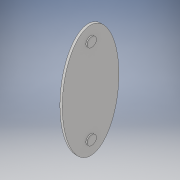
# Autodesk Inventor part: belt for lift
Saved by Autodesk Inventor 2017 (Build 210142000, 142)
## iProperties
Created: 2017-11-11
Part Number: belt for lift
Material: Generic
Document SubType Name: Modeling
Designer: User
Density: 1 g/cm^3
Appearance: Default
Author: User
Autodesk Inventor part; units mm, degrees
ref_plane "YZ Plane" through (0, 0, 0) normal (1, 0, 0) x (0, 1, 0)
ref_plane "XZ Plane" through (0, 0, 0) normal (0, 1, 0) x (-1, 0, 0)
ref_plane "XY Plane" through (0, 0, 0) normal (0, 0, 1) x (1, 0, 0)
sketch "Sketch1" plane through (0, 0, 0) normal (1, 0, 0) x (0, 1, 0)
  ellipse E0 centre (0, 0) end of major axis (76.2, 0) minor radius 38.1
  dimension "d0" = 38.1
  dimension "d1" = 76.2
  constraints: 1 coincident, 2 other
extrude "Extrusion1" add sketch "Sketch1" along normal blind 3.175
sketch "Sketch2" plane through (3.175, 0, 0) normal (1, 0, 0) x (0, 0, -1)
  ellipse E0 centre (0, 0) end of major axis (0, -76.2) minor radius 38.1 projected
  circle A0 centre (0, 57.15) radius 6.3627
  circle A1 centre (0, -57.15) radius 6.3627
  dimension "d4" = 57.15
  dimension "d5" = 57.15
  dimension "d6" = 12.7254
  dimension "d7" = 12.7254
  constraints: 2 centre point, 2 coincident, 1 other
  measures "d4" distance of point (0, 57.15) point (0, 0)
  measures "d5" distance of point (0, 0) point (0, -57.15)
  measures "d6" diameter of A0
  measures "d7" diameter of A1
extrude "Extrusion2" add sketch "Sketch2" along normal blind 1.5875 contours A0 | A1
equation "\"d7\" = d6"
body "Solid1"
